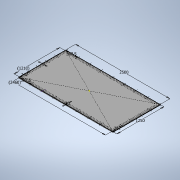
# Autodesk Inventor part: tabla
Saved by Autodesk Inventor 2021 (Build 250183000, 183)
## iProperties
Created: 2023-12-18
Part Number: tabla
Material: Generic
Document SubType Name: Modeling
Designer: assman
Density: 1 g/cm^3
Appearance: Default
Author: assman
Autodesk Inventor part; units mm, degrees
ref_plane "YZ Plane" through (0, 0, 0) normal (1, 0, 0) x (0, 1, 0)
ref_plane "XZ Plane" through (0, 0, 0) normal (0, 1, 0) x (-1, 0, 0)
ref_plane "XY Plane" through (0, 0, 0) normal (0, 0, 1) x (1, 0, 0)
sketch "Sketch1" plane through (0, 0, 0) normal (0, 1, 0) x (-1, 0, 0)
  line L0 (1250, 625) -> (-1250, 625)
  line L1 (-1250, 625) -> (-1250, -625)
  line L2 (-1250, -625) -> (1250, -625)
  line L3 (1250, -625) -> (1250, 625)
  line L4 (1250, 625) -> (-1250, -625) construction
  line L5 (-1250, 625) -> (1250, -625) construction
  line L6 (1210, 585) -> (-1210, 585) construction
  line L7 (-1210, 585) -> (-1210, -585) construction
  line L8 (-1210, -585) -> (1210, -585) construction
  line L9 (1210, -585) -> (1210, 585) construction
  line L10 (-1190, 565) -> (1190, 565) construction
  line L11 (1190, 565) -> (1190, -565) construction
  line L12 (1190, -565) -> (-1190, -565) construction
  line L13 (-1190, -565) -> (-1190, 565) construction
  line L14 (-1230, 605) -> (1230, 605) construction
  line L15 (1230, 605) -> (1230, -605) construction
  line L16 (1230, -605) -> (-1230, -605) construction
  line L17 (-1230, -605) -> (-1230, 605) construction
  point P0 (0, 0)
  point P1 (1230, 363)
  point P2 (1230, 121)
  point P3 (1230, -121)
  point P4 (1230, -363)
  point P5 (-1230, 363)
  point P6 (-1230, 121)
  point P7 (-1230, -121)
  point P8 (-1230, -363)
  point P9 (922.5, 605)
  point P10 (615, 605)
  point P11 (307.5, 605)
  point P12 (0, 605)
  point P13 (-307.5, 605)
  point P14 (-615, 605)
  point P15 (-922.5, 605)
  point P16 (922.5, -605)
  point P17 (615, -605)
  point P18 (307.5, -605)
  point P19 (0, -605)
  point P20 (-307.5, -605)
  point P21 (-615, -605)
  point P22 (-922.5, -605)
  point P23 (619.1026, 604.7999)
  dimension "d0" = 2500
  dimension "d1" = 1250
  dimension "d2" = 40
  dimension "d3" = 20
  dimension "d4" = 20
  dimension "d5" = 1210
  dimension "d6" = 2460
  dimension "d9" = 242
  dimension "d16" = 242
  dimension "d23" = 307.5
  dimension "d30" = 307.5
  constraints: 36 end point, 8 parallel, 4 perpendicular, 3 horizontal, 2 coincident, 2 midpoint, 2 vertical, 35 other
  measures "d0" distance of L2.end L1.end
  measures "d1" distance of L1.end L0.end
  measures "d2" distance between parallel lines of L3 L9
  measures "d3" distance between parallel lines of L6 L10
  measures "d4" distance between parallel lines of L0 L14
  measures "d5" distance of L14.end L15.end
  measures "d6" distance of L14.start L14.end
  measures "d9" distance of point (1230, 605) point (1230, 363)
  measures "d16" distance of point (-1230, 605) point (-1230, 363)
  measures "d23" distance of point (1230, 605) point (922.5, 605)
  measures "d30" distance of point (1230, -605) point (922.5, -605)
extrude "Extrusion1" add sketch "Sketch1" against normal blind 20
hole "Hole1" at (-1230, 0, 363) at (-1230, 0, 121) at (-1230, 0, -121) at (-1230, 0, -363) at (-1230, 0, -605) at (-922.5, 0, -605) at (-615, 0, -605) at (-307.5, 0, -605) at (0, 0, -605) at (307.5, 0, -605) at (615, 0, -605) at (922.5, 0, -605) at (1230, 0, -605) at (1230, 0, -363) at (1230, 0, -121) at (1230, 0, 121) at (1230, 0, 363) at (1230, 0, 605) at (922.5, 0, 605) at (615, 0, 605) at (307.5, 0, 605) at (0, 0, 605) at (-307.5, 0, 605) at (-922.5, 0, 605) at (-615, 0, 605) at (-1230, 0, 605) direction (0, -1, 0) diameter 10 end through all
body "Solid1"
